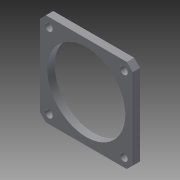
# Autodesk Inventor part: Cover Plate
Saved by Autodesk Inventor 2013 (Build 170138000, 138)
## iProperties
Created: 2014-11-16
Part Number: Cover Plate
Material: Generic
Document SubType Name: Modeling
Designer: Kyle
Density: 1 g/cm^3
Author: Kyle
Autodesk Inventor part; units mm, degrees
ref_plane "YZ Plane" through (0, 0, 0) normal (1, 0, 0) x (0, 1, 0)
ref_plane "XZ Plane" through (0, 0, 0) normal (0, 1, 0) x (-1, 0, 0)
ref_plane "XY Plane" through (0, 0, 0) normal (0, 0, 1) x (1, 0, 0)
sketch "Sketch1" plane through (0, 0, 0) normal (0, 0, 1) x (1, 0, 0)
  line L0 (0, 0) -> (40.005, 0)
  line L1 (40.005, 0) -> (40.005, -40.005)
  line L2 (40.005, -40.005) -> (0, -40.005)
  line L3 (0, -40.005) -> (0, 0)
  circle A0 centre (3.81, -36.195) radius 1.651
  circle A1 centre (3.81, -3.81) radius 1.651
  circle A2 centre (36.195, -36.195) radius 1.651
  circle A3 centre (36.195, -3.81) radius 1.651
  circle A4 centre (20.0025, -20.0025) radius 16.8275
  point P0 (20.0025, -3.175)
  point P1 (20.0025, -36.83)
  point P2 (36.83, -20.0025)
  point P3 (3.175, -20.0025)
  dimension "d0" = 40.005
  dimension "d1" = 40.005
  dimension "d2" = 3.175
  dimension "d3" = 3.175
  dimension "d4" = 3.175
  dimension "d5" = 3.175
  dimension "d6" = 3.81
  dimension "d7" = 3.81
  dimension "d8" = 3.81
  dimension "d9" = 3.81
  dimension "d10" = 3.302
  dimension "d11" = 3.302
  dimension "d13" = 3.302
  dimension "d14" = 3.302
  constraints: 8 end point, 4 centre point, 4 coincident, 2 parallel, 1 horizontal, 1 horizontal alignment, 1 perpendicular, 2 other
  measures "d0" distance of L0.start L0.end
  measures "d1" distance of L2.end L0.start
  measures "d2" distance from line of L3 point (3.175, -20.002)
  measures "d3" distance from line of L2 point (20.003, -36.83)
  measures "d4" distance from line of L1 point (36.83, -20.002)
  measures "d5" distance from line of L0 point (20.003, -3.175)
  measures "d6" distance from line of L2 point (36.195, -36.195)
  measures "d7" distance from line of point (36.195, -36.195) L1
  measures "d8" distance from line of L0 point (3.81, -3.81)
  measures "d9" distance from line of L3 point (3.81, -3.81)
  measures "d10" diameter of A0
  measures "d11" diameter of A1
  measures "d13" diameter of A2
  measures "d14" diameter of A3
extrude "Extrusion1" add sketch "Sketch1" along normal blind 3.175
chamfer "Chamfer1" distance 2.54 angle 45 4 edges at (0, 0, 1.5875) (40.005, 0, 1.5875) (40.005, -40.005, 1.5875) (0, -40.005, 1.5875)
body "Solid1"
